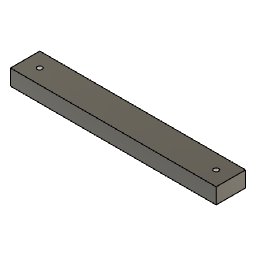
SupportAiments v2 (Autodesk Fusion 360 design; units mm, degrees)
Autodesk Fusion 360 part; units mm, degrees
box "BoitePrimitive1" add length 15 width 105.2 height 8 placed x (0, 1, 0) y (-1, 0, 0) z (0, 0, 1) at (115.2, 10, 0)
hole "Perçage1" at (17.5, 17.5, 8) direction (0, 0, -1) diameter 2.529 depth 6 tip angle 180
thread "Filetage1" "ISO Metric profile 3.0 M3x0.5 6H"
hole "Perçage2" at (107.7, 17.5, 8) direction (0, 0, -1) diameter 2.529 depth 6 tip angle 180
thread "Filetage2" "ISO Metric profile 3.0 M3x0.5 6H"
hole "Perçage3" at (28, 17.5, 0) direction (0, 0, 1) diameter 10.1 depth 2.2 tip angle 180
hole "Perçage4" at (97.2, 17.5, 0) direction (0, 0, 1) diameter 10.1 depth 2.2 tip angle 180
